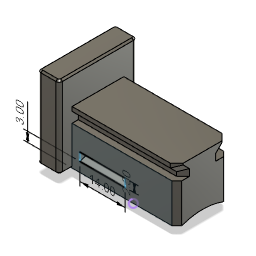
OBS-D-201_V1 (Autodesk Fusion 360 archive; units mm, degrees)
design "OBS-D-003VM"
Autodesk Fusion 360 part; units mm, degrees
sketch "Skizze1" plane through (0, 0, 0) normal (1, 0, 0) x (0, 0, -1)
  line L0 (-8, 5.2) -> (-6.05, 3.25)
  line L1 (-6.05, 3.25) -> (-6.05, 2)
  line L2 (6.05, 2) -> (6.05, 3.25)
  line L3 (6.05, 3.25) -> (8, 5.2)
  line L4 (8, 5.2) -> (8, 6.5)
  line L5 (8, 6.5) -> (-8, 6.5)
  line L6 (-8, 6.5) -> (-8, 5.2)
  line L7 (-6.05, 2) -> (-8, 2)
  line L8 (-8, 2) -> (-8, 0)
  line L9 (-8, 0) -> (8, 0)
  line L10 (8, 0) -> (8, 2)
  line L11 (8, 2) -> (6.05, 2)
  line L12 (0, 6.5) -> (0, 0) construction
  dimension "d5" = 16
  dimension "d6" = 1.3
  dimension "d8" = 2
  dimension "d26" = 12.1
  dimension "d27" = 4.5
  dimension "d28" = 135
  constraint vertical L1
  constraint perpendicular L2 L5
  constraint perpendicular L5 L6
  constraint vertical L4
  constraint perpendicular L1 L7
  constraint perpendicular L7 L8
  constraint perpendicular L8 L9
  constraint perpendicular L7 L10
  constraint perpendicular L2 L11
  constraint collinear L4 L10
  constraint collinear L6 L8
  constraint midpoint L5 L12.start
  constraint midpoint L9 L12.end
  constraint symmetric L0.start L3.end L12
  constraint symmetric L0.end L2.end L12
  constraint midpoint L12.end L9
  constraint collinear L7 L11
  measures "d5" distance of L4.end L5.end
  measures "d6" distance of L0.start L5.end
  measures "d8" distance of L7 L9
  measures "d26" distance of L1 L2
  measures "d27" distance of L5 L7
  measures "d28" angle of L0 L6
extrude "Extrusion1" add sketch "Skizze1" along normal blind 32.4 makes body 1
sketch "Skizze7" plane through (0, 0, 0) normal (0, 1, 0) x (1, 0, 0)
  line L0 (0, -12) -> (-6.6, -12)
  line L1 (-6.6, -12) -> (-6.6, 12)
  line L2 (-6.6, 12) -> (0, 12)
  line L3 (0, 12) -> (0, -12)
  line L4 (-0.8, -10) -> (-4.6, -10)
  line L5 (-4.6, -10) -> (-4.6, 10)
  line L6 (-4.6, 10) -> (-0.8, 10)
  line L7 (-0.8, 10) -> (-0.8, -10)
  line L8 (0, 0) -> (-0.8, 0) construction
  line L9 (-2.7, -10) -> (-2.7, 10)
  dimension "d82" = 24
  dimension "d83" = 0.8
  dimension "d84" = 2
  dimension "d85" = 3.8
  dimension "d86" = 20
  constraint horizontal L0
  constraint vertical L1
  constraint horizontal L2
  constraint vertical L3
  constraint midpoint L8.start L3
  constraint horizontal L4
  constraint vertical L5
  constraint horizontal L6
  constraint vertical L7
  constraint coincident L8.start origin
  constraint midpoint L7 L8.end
  constraint horizontal L8
  constraint midpoint L4 L9.start
  constraint midpoint L6 L9.end
  measures "d82" distance of L0.start L2.end
  measures "d83" distance of L3 L7
  measures "d84" distance of L1 L5
  measures "d85" distance of L5 L7
  measures "d86" distance of L4.end L5.end
extrude "Extrusion17" add sketch "Skizze7" along normal blind 21.2 bodies 1
extrude "Extrusion18" add sketch "Skizze7" along normal blind 15.2 contours L4 L6 L7 L9 | L4 L5 L6 L9 bodies 1
extrude "Extrusion19" add sketch "Skizze7" against normal blind 1.5 from surface at 21.2 contours L4 L6 L7 L9 bodies 1
sketch "Skizze3" plane through (0, 0, 0) normal (1, 0, 0) x (0, 0, -1)
  circle A0 centre (0.0294, -25) radius 17
  line L0 (24, -24) -> (24, 0)
  line L1 (24, 0) -> (-23.9411, 0)
  line L2 (-23.9411, 0) -> (-23.9411, -24)
  line L3 (17, -24) -> (-16.9411, -24) construction
  line L4 (17, -24) -> (24, -24)
  line L5 (-16.9411, -24) -> (-23.9411, -24)
  line L6 (17, -26) -> (-16.9411, -26) construction
  line L7 (17, -26) -> (24, -26)
  line L8 (24, -26) -> (24, -46)
  line L9 (24, -46) -> (-23.9411, -46)
  line L10 (-23.9411, -46) -> (-23.9411, -26)
  line L11 (-23.9411, -26) -> (-16.9411, -26)
  line L12 (0.0294, -25) -> (0.0294, -8) construction
  line L13 (0.0294, -42) -> (0.0294, -25) construction
  circle A1 centre (0.0294, -25) radius 16.8
  line L14 (17, -24) -> (-16.7408, -24)
  line L15 (17, -26) -> (-16.7408, -26)
  line L16 (-16.9411, -24) -> (16.7996, -24)
  line L17 (-16.9411, -26) -> (16.7996, -26)
  dimension "d29" = 34
  dimension "d30" = 7
  dimension "d31" = 7
  dimension "d32" = 24
  dimension "d33" = 1
  dimension "d34" = 1
  dimension "d35" = 8
  dimension "d37" = 4
  dimension "d111" = 33.6
  constraint coincident A0 L3.start
  constraint coincident A0 L3.end
  constraint horizontal L3
  constraint horizontal L4
  constraint horizontal L5
  constraint vertical L0
  constraint coincident A0 L6.start
  constraint coincident A0 L6.end
  constraint horizontal L6
  constraint perpendicular L0 L7
  constraint perpendicular L10 L11
  constraint coincident A0.centre L12.start
  constraint coincident A0 L12.end
  constraint vertical L12
  constraint horizontal L1
  constraint vertical L2
  constraint vertical L8
  constraint horizontal L9
  constraint vertical L10
  constraint collinear L2 L10
  constraint collinear L0 L8
  constraint coincident A0 L13.start
  constraint perpendicular L6 L13
  constraint coincident origin L1
  constraint coincident A1 L14.end
  constraint coincident L3 L14.end
  constraint coincident A1 L15.end
  constraint coincident L6 L15.end
  constraint coincident A1 L16.end
  constraint coincident L3 L16.end
  constraint coincident A1 L17.end
  constraint coincident L6 L17.end
  measures "d29" diameter of A0
  measures "d30" distance of L0.start L3.start
  measures "d31" distance of L2.end L3.end
  measures "d32" distance of origin L0
  measures "d33" distance of A0.centre L3
  measures "d34" distance of A0.centre L6
  measures "d35" vertical distance of origin L12.end
  measures "d37" distance of L9 L13.start
  measures "d111" diameter of A1
extrude "Extrusion6" [suppressed]
extrude "Extrusion23" [suppressed]
chamfer "Fase1" [suppressed]
chamfer "Fase2" [suppressed]
fillet "Abrundung1" [suppressed]
ref_plane "Arbeitsebene1" through (0, -9, 0) normal (0, 1, 0) x (0, 0, 1)
sketch "Skizze4" plane through (0, -9, 0) normal (0, 1, 0) x (1, 0, 0)
  line L0 (0, 0.0294) -> (5, 0.0294) construction
  line L1 (3.4, 19.1294) -> (3.4, -19.0706)
  arc A0 (3.4, -19.0706) -> (6.6, -19.0706) centre (5, -19.0706) ccw
  line L2 (6.6, -19.0706) -> (6.6, 19.1294)
  arc A1 (6.6, 19.1294) -> (3.4, 19.1294) centre (5, 19.1294) ccw
  line L3 (5, 19.1294) -> (5, -19.0706) construction
  arc A2 (6.6, -19.0706) -> (3.4, -19.0706) centre (5, -19.0706) ccw
  arc A3 (3.4, 19.1294) -> (6.6, 19.1294) centre (5, 19.1294) ccw
  line L4 (7.75, 19.1294) -> (7.75, 27.1294)
  arc A4 (7.75, 27.1294) -> (2.25, 27.1294) centre (5, 27.1294) ccw
  line L5 (2.25, 27.1294) -> (2.25, 19.1294)
  arc A5 (2.25, 19.1294) -> (7.75, 19.1294) centre (5, 19.1294) ccw
  line L6 (5, 19.1294) -> (5, 27.1294) construction
  line L7 (2.25, -19.0706) -> (2.25, -27.0706)
  arc A6 (2.25, -27.0706) -> (7.75, -27.0706) centre (5, -27.0706) ccw
  line L8 (7.75, -27.0706) -> (7.75, -19.0706)
  arc A7 (7.75, -19.0706) -> (2.25, -19.0706) centre (5, -19.0706) ccw
  line L9 (5, -19.0706) -> (5, -27.0706) construction
  line L10 (12.5, 16.976) -> (12.5, -37.3443) construction
  arc A8 (22.75, 27.1294) -> (17.25, 27.1294) centre (20, 27.1294) ccw
  line L11 (17.25, 19.1294) -> (17.25, 27.1294)
  line L12 (18.4, -19.0706) -> (18.4, 19.1294)
  arc A9 (21.6, -19.0706) -> (18.4, -19.0706) centre (20, -19.0706) ccw
  line L13 (17.25, -27.0706) -> (17.25, -19.0706)
  arc A10 (21.6, 19.1294) -> (18.4, 19.1294) centre (20, 19.1294) ccw
  arc A11 (17.25, -27.0706) -> (22.75, -27.0706) centre (20, -27.0706) ccw
  arc A12 (22.75, -19.0706) -> (17.25, -19.0706) centre (20, -19.0706) ccw
  line L14 (22.75, 27.1294) -> (22.75, 19.1294)
  line L15 (20, 19.1294) -> (20, -19.0706) construction
  arc A13 (18.4, -19.0706) -> (21.6, -19.0706) centre (20, -19.0706) ccw
  line L16 (20, -19.0706) -> (20, -27.0706) construction
  line L17 (22.75, -19.0706) -> (22.75, -27.0706)
  line L18 (20, 19.1294) -> (20, 27.1294) construction
  arc A14 (18.4, 19.1294) -> (21.6, 19.1294) centre (20, 19.1294) ccw
  line L19 (21.6, 19.1294) -> (21.6, -19.0706)
  arc A15 (17.25, 19.1294) -> (22.75, 19.1294) centre (20, 19.1294) ccw
  line L20 (2.25, 20.7294) -> (7.75, 20.7294)
  line L21 (6.6, 20.7294) -> (6.6, 17.5294)
  line L22 (7.2366, 17.5294) -> (2.7634, 17.5294)
  line L23 (3.4, 17.5294) -> (3.4, 20.7294)
  line L24 (17.25, 20.7294) -> (22.75, 20.7294)
  line L25 (21.6, 20.7294) -> (21.6, 17.5294)
  line L26 (22.2366, 17.5294) -> (17.7634, 17.5294)
  line L27 (18.4, 17.5294) -> (18.4, 20.7294)
  line L28 (2.7634, -17.4706) -> (7.2366, -17.4706)
  line L29 (6.6, -17.4706) -> (6.6, -20.6706)
  line L30 (7.75, -20.6706) -> (2.25, -20.6706)
  line L31 (3.4, -20.6706) -> (3.4, -17.4706)
  line L32 (17.7634, -17.4706) -> (22.2366, -17.4706)
  line L33 (21.6, -17.4706) -> (21.6, -20.6706)
  line L34 (22.75, -20.6706) -> (17.25, -20.6706)
  line L35 (18.4, -20.6706) -> (18.4, -17.4706)
  line L36 (0, 16.7996) -> (25, 16.7996)
  point P0 (0, 0.0294)
  point P1 (5, 0.0294)
  point P2 (5, -17.4706)
  point P3 (20, 0.0294)
  point P4 (20, 0.0294)
  point P5 (20, -17.4706)
  dimension "d43" = 5
  dimension "d44" = 1.6
  dimension "d46" = 5.5
  dimension "d47" = 5.5
  dimension "d48" = 8
  dimension "d49" = 8
  dimension "d59" = 12.5
  dimension "d117" = 17.5
  constraint horizontal L0
  constraint tangent L1 A0
  constraint tangent A0 L2
  constraint parallel L1 L2
  constraint tangent L2 A1
  constraint tangent L1 A1
  constraint perpendicular L0 L3
  constraint coincident P1 L0.end
  constraint midpoint L3 P1
  constraint tangent L1 A2
  constraint tangent L2 A3
  constraint midpoint A2 P2
  constraint tangent L4 A4
  constraint tangent A4 L5
  constraint parallel L4 L5
  constraint tangent L5 A5
  constraint tangent L4 A5
  constraint parallel L3 L6
  constraint coincident A1.centre L3.start
  constraint tangent L7 A6
  constraint tangent A6 L8
  constraint parallel L7 L8
  constraint tangent L8 A7
  constraint tangent L7 A7
  constraint parallel L3 L9
  constraint coincident A0.centre L3.end
  constraint vertical L10
  constraint symmetric P1 L10 P4
  constraint symmetric L1.start L10 A10.start
  constraint symmetric L1.end L10 A9.start
  constraint symmetric A0.end L10 L12.start
  constraint symmetric L2.end L10 L12.end
  constraint symmetric A0 L10 A13
  constraint symmetric A1 L10 A10
  constraint symmetric A2 L10 A9
  constraint symmetric A3 L10 A14
  constraint symmetric P2 L10 P5
  constraint symmetric L4.start L10 L11.start
  constraint symmetric L4.end L10 A8.end
  constraint symmetric A4.end L10 A8.start
  constraint symmetric L5.end L10 L14.end
  constraint symmetric A4 L10 A8
  constraint symmetric A5 L10 A15
  constraint symmetric L7.start L10 A12.start
  constraint symmetric L7.end L10 A11.end
  constraint symmetric A6.end L10 L13.start
  constraint symmetric L8.end L10 L13.end
  constraint symmetric A6 L10 A11
  constraint symmetric A7 L10 A12
  constraint horizontal L20
  constraint vertical L21
  constraint horizontal L22
  constraint vertical L23
  constraint horizontal L24
  constraint vertical L25
  constraint horizontal L26
  constraint vertical L27
  constraint horizontal L28
  constraint vertical L29
  constraint horizontal L30
  constraint vertical L31
  constraint horizontal L32
  constraint vertical L33
  constraint horizontal L34
  constraint vertical L35
  constraint tangent A0 L29
  constraint tangent A2 L28
  constraint tangent A2 L31
  constraint tangent A0 L30
  constraint tangent A13 L33
  constraint tangent A9 L32
  constraint tangent A13 L35
  constraint tangent A13 L34
  constraint tangent A10 L25
  constraint tangent A10 L27
  constraint tangent A10 L24
  constraint tangent A14 L26
  constraint tangent A3 L22
  constraint tangent A3 L21
  constraint tangent A1 L23
  constraint tangent A1 L20
  constraint coincident L4 L20.end
  constraint coincident L21.start L20
  constraint coincident A5 L22.start
  constraint coincident L21.end L22
  constraint coincident A5 L22.end
  constraint coincident L23.start L22
  constraint coincident L5 L20.start
  constraint coincident L23.end L20
  constraint coincident L11 L24.start
  constraint coincident L27.end L24
  constraint coincident A15 L26.end
  constraint coincident L27.start L26
  constraint coincident A15 L26.start
  constraint coincident L25.end L26
  constraint coincident L14 L24.end
  constraint coincident L25.start L24
  constraint coincident A12 L32.start
  constraint coincident L35.end L32
  constraint coincident A12 L32.end
  constraint coincident L33.start L32
  constraint coincident L33.end L34
  constraint coincident L35.start L34
  constraint coincident A7 L28.end
  constraint coincident L29.start L28
  constraint coincident L29.end L30
  constraint coincident L31.start L30
  constraint coincident A7 L28.start
  constraint coincident L31.end L28
  constraint coincident P0 L0
  constraint coincident P0 L0.start
  measures "d43" distance of P0 P1
  measures "d44" radius of A0
  measures "d46" distance of L4 L5
  measures "d47" distance of L7 L8
  measures "d48" distance of A1.centre A4.centre
  measures "d49" distance of A0.centre A6.centre
  measures "d59" distance of P0 L10
  measures "d117" distance of P4 L22
extrude "Extrusion7" [suppressed]
extrude "Extrusion8" [suppressed]
extrude "Extrusion9" [suppressed]
extrude "Extrusion13" [suppressed]
extrude "Extrusion14" [suppressed]
ref_plane "Arbeitsebene2" through (0, -33, 0) normal (0, 1, 0) x (0, 0, 1)
sketch "Skizze5" plane through (0, -33, 0) normal (0, 1, 0) x (1, 0, 0)
  arc A0 (21.6, 19.1294) -> (18.4, 19.1294) centre (20, 19.1294) ccw
  arc A1 (6.6, 19.1294) -> (3.4, 19.1294) centre (5, 19.1294) ccw
  arc A2 (3.4, -19.0706) -> (6.6, -19.0706) centre (5, -19.0706) ccw
  arc A3 (18.4, -19.0706) -> (21.6, -19.0706) centre (20, -19.0706) ccw
  line L0 (2.2, 17.5129) -> (5, 15.8963)
  line L1 (5, 15.8963) -> (7.8, 17.5129)
  line L2 (7.8, 17.5129) -> (7.8, 20.746)
  line L3 (7.8, 20.746) -> (5, 22.3626)
  line L4 (5, 22.3626) -> (2.2, 20.746)
  line L5 (2.2, 20.746) -> (2.2, 17.5129)
  line L6 (2.2, -20.6871) -> (5, -22.3037)
  line L7 (5, -22.3037) -> (7.8, -20.6871)
  line L8 (7.8, -20.6871) -> (7.8, -17.454)
  line L9 (7.8, -17.454) -> (5, -15.8374)
  line L10 (5, -15.8374) -> (2.2, -17.454)
  line L11 (2.2, -17.454) -> (2.2, -20.6871)
  line L12 (17.2, -20.6871) -> (20, -22.3037)
  line L13 (20, -22.3037) -> (22.8, -20.6871)
  line L14 (22.8, -20.6871) -> (22.8, -17.454)
  line L15 (22.8, -17.454) -> (20, -15.8374)
  line L16 (20, -15.8374) -> (17.2, -17.454)
  line L17 (17.2, -17.454) -> (17.2, -20.6871)
  line L18 (17.2, 17.5129) -> (20, 15.8963)
  line L19 (20, 15.8963) -> (22.8, 17.5129)
  line L20 (22.8, 17.5129) -> (22.8, 20.746)
  line L21 (22.8, 20.746) -> (20, 22.3626)
  line L22 (20, 22.3626) -> (17.2, 20.746)
  line L23 (17.2, 20.746) -> (17.2, 17.5129)
  arc A4 (21.6, -19.0706) -> (18.4, -19.0706) centre (20, -19.0706) ccw
  arc A5 (6.6, -19.0706) -> (3.4, -19.0706) centre (5, -19.0706) ccw
  arc A6 (3.4, 19.1294) -> (6.6, 19.1294) centre (5, 19.1294) ccw
  arc A7 (18.4, 19.1294) -> (21.6, 19.1294) centre (20, 19.1294) ccw
  line L24 (2.2, -20.6871) -> (7.8, -20.6871)
  line L25 (7.8, -17.454) -> (2.2, -17.454)
  line L26 (17.2, -20.6871) -> (22.8, -20.6871)
  line L27 (22.8, -17.454) -> (17.2, -17.454)
  line L28 (7.8, 17.5129) -> (2.2, 17.5129)
  line L29 (2.2, 20.746) -> (7.8, 20.746)
  line L30 (17.2, 20.746) -> (22.8, 20.746)
  line L31 (22.8, 17.5129) -> (17.2, 17.5129)
  line L32 (21.6, 17.5129) -> (21.6, 10.2479)
  line L33 (18.4, 17.5129) -> (18.4, 20.746)
  line L34 (3.4, 17.5129) -> (3.4, 20.746)
  line L35 (6.6, 20.746) -> (6.6, 17.5129)
  line L36 (3.4, -20.6871) -> (3.4, -17.454)
  line L37 (6.6, -17.454) -> (6.6, -20.6871)
  line L38 (18.4, -20.6871) -> (18.4, -17.454)
  line L39 (21.6, -20.6871) -> (21.6, -17.454)
  point P0 (5, 19.1294)
  point P1 (20, 19.1294)
  point P2 (20, -19.0706)
  point P3 (5, -19.0706)
  point P4 (5, 19.1294)
  point P5 (5, -19.0706)
  point P6 (20, -19.0706)
  point P7 (20, 19.1294)
  dimension "d61" = 5.6
  constraint coincident P4 P0
  constraint coincident P5 P3
  constraint coincident P6 P2
  constraint coincident P7 P1
  constraint equal L2 L23
  constraint equal L2 L8
  constraint equal L8 L17
  constraint vertical L5
  constraint vertical L23
  constraint vertical L17
  constraint vertical L11
  constraint coincident L31 L32.start
  constraint perpendicular L31 L32
  constraint coincident L31 L33.start
  constraint coincident L30 L33.end
  constraint perpendicular L30 L33
  constraint coincident L28 L34.start
  constraint coincident L29 L34.end
  constraint perpendicular L29 L34
  constraint coincident L29 L35.start
  constraint coincident L28 L35.end
  constraint perpendicular L28 L35
  constraint tangent A7 L32
  constraint tangent A7 L33
  constraint tangent A6 L35
  constraint tangent A6 L34
  constraint coincident L24 L36.start
  constraint coincident L25 L36.end
  constraint perpendicular L25 L36
  constraint coincident L25 L37.start
  constraint coincident L24 L37.end
  constraint perpendicular L24 L37
  constraint coincident L26 L38.start
  constraint coincident L27 L38.end
  constraint perpendicular L27 L38
  constraint coincident L26 L39.start
  constraint coincident L27 L39.end
  constraint perpendicular L27 L39
  constraint tangent A2 L36
  constraint tangent A2 L37
  constraint tangent A3 L38
  constraint tangent A3 L39
  measures "d61" distance of L2 L5
extrude "Extrusion10" [suppressed]
extrude "Extrusion11" [suppressed]
extrude "Extrusion12" [suppressed]
sketch "Skizze6" plane through (0, 0, 0) normal (0, 1, 0) x (1, 0, 0)
  line L0 (0, 0) -> (0.2903, 0)
  line L1 (0.2903, 0) -> (23.3187, 0) construction
  circle A0 centre (5, 0) radius 1.6
  circle A1 centre (20, 0) radius 1.6
  line L2 (22.8, 1.6166) -> (20, 3.2332)
  line L3 (20, 3.2332) -> (17.2, 1.6166)
  line L4 (17.2, 1.6166) -> (17.2, -1.6166)
  line L5 (17.2, -1.6166) -> (20, -3.2332)
  line L6 (20, -3.2332) -> (22.8, -1.6166)
  line L7 (22.8, -1.6166) -> (22.8, 1.6166)
  line L8 (7.8, 1.6166) -> (5, 3.2332)
  line L9 (5, 3.2332) -> (2.2, 1.6166)
  line L10 (2.2, 1.6166) -> (2.2, -1.6166)
  line L11 (2.2, -1.6166) -> (5, -3.2332)
  line L12 (5, -3.2332) -> (7.8, -1.6166)
  line L13 (7.8, -1.6166) -> (7.8, 1.6166)
  point P0 (20, 0)
  point P1 (5, 0)
  dimension "d72" = 20
  dimension "d73" = 5
  dimension "d74" = 3.2
  dimension "d75" = 5.6
  constraint coincident L0.start origin
  constraint horizontal L0
  constraint parallel L0 L1
  constraint coincident L1 P1
  constraint coincident L1 P0
  constraint equal A0 A1
  constraint coincident P0 A1.centre
  constraint coincident P1 A0.centre
  constraint equal L4 L13
  constraint vertical L13
  constraint vertical L4
  measures "d72" distance of L0.start A1.centre
  measures "d73" distance of L0.start P1
  measures "d74" diameter of A0
  measures "d75" distance of L4 L7
extrude "Extrusion15" [suppressed]
extrude "Extrusion16" [suppressed]
sketch "Skizze9" plane through (0, 6.5, 0) normal (0, 1, 0) x (-1, 0, 0)
  line L0 (0, -8) -> (0, 8)
  line L1 (0, 8) -> (-37, 8)
  line L2 (-37, 8) -> (-37, -8)
  line L3 (-37, -8) -> (0, -8)
  circle A0 centre (-5, 0) radius 1.6
  circle A1 centre (-20, 0) radius 1.6
  circle A2 centre (-20, 0) radius 3
  circle A3 centre (-5, 0) radius 3
  dimension "d94" = 6
  constraint concentric A1 A2
  constraint concentric A0 A3
  constraint equal A2 A3
  measures "d94" diameter of A2
extrude "Extrusion20" [suppressed]
extrude "Extrusion21" [suppressed]
fillet "Abrundung2" [suppressed]
move_face "Flächen versetzen1" offset 10 1 faces at (21.6, 0, 2.6667) on bodies 1
sketch "Skizze10" plane through (0, -10, 0) normal (0, -1, 0) x (1, 0, 0)
  line L0 (0, -8) -> (32.4, -8)
  line L1 (32.4, -8) -> (32.4, 8)
  line L2 (32.4, 8) -> (0, 8)
  line L3 (0, 8) -> (0, 12)
  line L4 (0, 12) -> (-6.6, 12)
  line L5 (-6.6, 12) -> (-6.6, -12)
  line L6 (-6.6, -12) -> (0, -12)
  line L7 (0, -12) -> (0, -8)
  line L8 (29.8, 8) -> (-5.1, 8)
  line L9 (18.949, -2.45) -> (28.949, -2.45)
  line L10 (18.949, 2.55) -> (18.949, -2.45)
  line L11 (28.949, 2.55) -> (18.949, 2.55)
  line L12 (28.949, 2.55) -> (29.8, 2.55) construction
  line L13 (28.949, -2.45) -> (28.949, 2.55)
  line L14 (29.8, -8) -> (29.8, 8)
  point P0 (29.8, 4.05)
  point P1 (35.1346, -3.1735)
  dimension "d119" = 10
  dimension "d120" = 5
  dimension "d121" = 1.5
  dimension "d125" = 5.45
  dimension "d126" = 5.45
  dimension "d130" = 25.549
  constraint horizontal L11
  constraint vertical L10
  constraint horizontal L9
  constraint vertical L13
  constraint coincident L12.end L14
  constraint perpendicular L12 L14
  measures "d119" distance of L11.start L10.start
  measures "d120" distance of L11.start L9.end
  measures "d121" distance of P0 L12.end
  measures "d125" distance of L8 L11
  measures "d126" distance of L2 L11
  measures "d130" distance of L5 L10
extrude "Extrusion24" cut sketch "Skizze10" against normal blind 15.1 contours L9 L10 L11 L13 bodies 1
fillet "Abrundung3" radius 1 4 edges at (0, 10.6, -12) (-6.6, 10.6, -12) (0, 10.6, 12) (-6.6, 10.6, 12) on bodies 1
chamfer "Fase3" distance 0.5 angle 45 9 edges at (0, -10, -9.5) (-0.2929, -10, -11.7071) (-3.3, -10, -12) (-6.3071, -10, -11.7071) (-6.6, -10, 0) (-6.3071, -10, 11.7071) (-3.3, -10, 12) (-0.2929, -10, 11.7071) (0, -10, 9.5) on bodies 1
chamfer "Fase4" distance 2 angle 45 6 edges at (32.4, 2.625, -6.05) (32.4, 2.625, 6.05) (32.4, 5.85, 8) (32.4, 5.85, -8) (32.4, 4.225, 7.025) (32.4, 4.225, -7.025) on bodies 1
extrude "Extrusion22" [suppressed]
chamfer "Fase5" [suppressed]
chamfer "Fase6" [suppressed]
chamfer "Fase7" distance 1.5 angle 45 2 edges at (32.4, 1, 8) (32.4, 1, -8) on bodies 1
sketch "Skizze11" plane through (0, 0, 8) normal (0, 0, 1) x (1, 0, 0)
  line L0 (30.9, -10) -> (30.9, 2)
  line L1 (30.9, 2) -> (0, 2)
  line L2 (0, 2) -> (0, -9.5)
  line L3 (0, -9.5) -> (-0.5, -10)
  line L4 (-0.5, -10) -> (30.9, -10)
  line L5 (2.4407, -4.5) -> (16.4407, -4.5)
  line L6 (16.4407, -4.5) -> (16.4407, -7)
  line L7 (16.4407, -7) -> (2.4407, -7)
  line L8 (2.4407, -7) -> (2.4407, -4.5)
  point P0 (18.949, -10)
  dimension "d136" = 2.5
  dimension "d137" = 3
  dimension "d152" = 14
  constraint horizontal L5
  constraint vertical L6
  constraint horizontal L7
  constraint vertical L8
  measures "d136" distance of L5.end L6.end
  measures "d137" distance of L4 L7
  measures "d152" distance of L6.end L7.end
sketch "Skizze12" plane through (32.4, 0, 0) normal (1, 0, 0) x (0, 0, -1)
  line L0 (6.5, -10) -> (6.5, 2)
  line L1 (6.5, 2) -> (4.05, 2)
  line L2 (4.05, 2) -> (4.05, 4.0784)
  line L3 (4.05, 4.0784) -> (6, 6.0284)
  line L4 (6, 6.0284) -> (6, 6.5)
  line L5 (6, 6.5) -> (-6, 6.5)
  line L6 (-6, 6.5) -> (-6, 6.0284)
  line L7 (-6, 6.0284) -> (-4.05, 4.0784)
  line L8 (-4.05, 4.0784) -> (-4.05, 2)
  line L9 (-4.05, 2) -> (-6.5, 2)
  line L10 (-6.5, 2) -> (-6.5, -10)
  line L11 (-6.5, -10) -> (6.5, -10)
  line L12 (0, 6.8761) -> (0, -26.8761) construction
  line L13 (-6.5, -10) -> (6.5, -10) construction
  circle A0 centre (0, -26.8761) radius 18
  circle A1 centre (0, -20.0295) radius 11.1
  dimension "d132" = 36
  dimension "d153" = 22.2
  constraint perpendicular L11 L12
  constraint midpoint L12 L13
  constraint coincident L12.end A0.centre
  constraint coincident L12 A1.centre
  measures "d132" diameter of A0
  measures "d153" diameter of A1
extrude "Extrusion25" cut sketch "Skizze12" against normal blind 46 contours L11 A0 A1 | L11 A1 picked at (4.9415, -9.7611) picked at (1.0764, -9.8032) bodies 1
ref_plane "Arbeitsebene3" through (6.4, -1.75, 0) normal (1, 0, 0) x (0, 0, -1)
sketch "Skizze13" plane through (6.4, -1.75, 0) normal (1, 0, 0) x (0, 1, 0)
  circle A0 centre (-25.1261, 0) radius 20.0974
  circle A1 centre (-24.0351, -0.1251) radius 18.8725
  circle A2 centre (-18.2795, 0) radius 11.1
  circle A3 centre (-16.7075, -0.2233) radius 12.2402
  point P0 (-25.1261, 0)
  constraint coincident P0 A0.centre
sweep "Sweeping1" cut profiles "Skizze11" path "Skizze13" along A0 section 1 contours L5 L6 L7 L8 bodies 1
extrude "Extrusion26" add sketch "Skizze12" along normal mid plane 230 separate body contours L11 A0 A1 | L11 A0 A1 | L11 A1 | L11 A1 makes body 3
sweep "Sweeping2" add profiles "Skizze11" path "Skizze13" along A1 section 1 contours L5 L6 L7 L8 separate body makes body 4
extrude "Extrusion27" add sketch "Skizze12" along normal mid plane 360 separate body contours L11 A1 | L11 A1 makes body 5
sweep "Sweeping3" add profiles "Skizze11" path "Skizze13" along A3 section 1 contours L5 L6 L7 L8 separate body makes body 6
extrude "Extrusion28" cut 1 faces at (-0.9, 21.2, -3.3333) along direction (0, -1, 0) blind 6 on bodies 1 bodies 1
chamfer "Fase8" distance 0.5 angle 45 8 edges at (-3.3, 15.2, 12) (-6.3071, 15.2, 11.7071) (-6.6, 15.2, 0) (-6.3071, 15.2, -11.7071) (-3.3, 15.2, -12) (-0.2929, 15.2, -11.7071) (0, 15.2, 0) (-0.2929, 15.2, 11.7071) on bodies 1
hidden bodies 3 4 5 6
equation "d9 = 37 mm - 4.6 mm"
equation "d72 = 25 mm - 5 mm"
equation "d87 = 9.7 mm + 10 mm + 1.5 mm"
equation "d89 = 9.7 mm + 5.5 mm"
equation "d117 = ( 32 / 2 ) * 1 mm + 1.5 mm"
equation "d126 = d125"
equation "d130 = 30.149028 mm - 4.6 mm"
